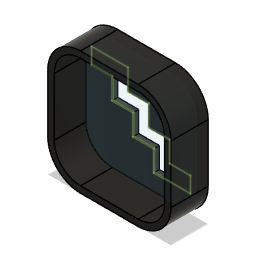
Trellis Keycap stairs (Autodesk Fusion 360 design; units mm, degrees)
Autodesk Fusion 360 part; units mm, degrees
sketch "Sketch1" plane through (0, 0, 0) normal (0, 0, 1) x (1, 0, 0)
  line L0 (2.72, 5) -> (-2.72, 5)
  line L1 (-5, 2.72) -> (-5, -2.72)
  line L2 (-2.72, -5) -> (2.72, -5)
  line L3 (5, -2.72) -> (5, 2.72)
  line L4 (5, 5) -> (-5, -5) construction
  line L5 (-5, 5) -> (5, -5) construction
  arc A0 (5, 2.72) -> (2.72, 5) centre (2.72, 2.72) ccw
  arc A1 (2.72, -5) -> (5, -2.72) centre (2.72, -2.72) ccw
  arc A2 (-5, -2.72) -> (-2.72, -5) centre (-2.72, -2.72) ccw
  arc A3 (-2.72, 5) -> (-5, 2.72) centre (-2.72, 2.72) ccw
  line L6 (-2.72, -5.2) -> (2.72, -5.2)
  arc A4 (2.72, -5.2) -> (5.2, -2.72) centre (2.72, -2.72) ccw
  line L7 (5.2, -2.72) -> (5.2, 2.72)
  arc A5 (5.2, 2.72) -> (2.72, 5.2) centre (2.72, 2.72) ccw
  line L8 (2.72, 5.2) -> (-2.72, 5.2)
  arc A6 (-2.72, 5.2) -> (-5.2, 2.72) centre (-2.72, 2.72) ccw
  line L9 (-5.2, 2.72) -> (-5.2, -2.72)
  arc A7 (-5.2, -2.72) -> (-2.72, -5.2) centre (-2.72, -2.72) ccw
  line L10 (-2.72, -5.8) -> (2.72, -5.8)
  arc A8 (2.72, -5.8) -> (5.8, -2.72) centre (2.72, -2.72) ccw
  line L11 (5.8, -2.72) -> (5.8, 2.72)
  arc A9 (5.8, 2.72) -> (2.72, 5.8) centre (2.72, 2.72) ccw
  line L12 (2.72, 5.8) -> (-2.72, 5.8)
  arc A10 (-2.72, 5.8) -> (-5.8, 2.72) centre (-2.72, 2.72) ccw
  line L13 (-5.8, 2.72) -> (-5.8, -2.72)
  arc A11 (-5.8, -2.72) -> (-2.72, -5.8) centre (-2.72, -2.72) ccw
  dimension "d1" = 10
  dimension "d2" = 10
  dimension "d3" = 2.28
  dimension "d4" = 0.2
  dimension "d5" = 0.8
  constraint horizontal L0
  constraint perpendicular L0 L1
  constraint parallel L0 L2
  constraint parallel L1 L3
  constraint coincident L4 origin
  constraint coincident L5 origin
  constraint coincident L4.start L0
  constraint coincident L4.start L3
  constraint tangent L0 A0
  constraint tangent L3 A0
  constraint coincident L5.end L3
  constraint coincident L5.end L2
  constraint tangent L3 A1
  constraint tangent L2 A1
  constraint equal A0 A1
  constraint coincident L4.end L2
  constraint coincident L4.end L1
  constraint tangent L2 A2
  constraint tangent L1 A2
  constraint equal A0 A2
  constraint coincident L5.start L1
  constraint coincident L5.start L0
  constraint tangent L1 A3
  constraint tangent L0 A3
  constraint equal A0 A3
  measures "d1" distance of L4.end L5.end
  measures "d2" distance of L5.start L4.end
  measures "d3" radius of A0
extrude "Extrude1" add sketch "Sketch1" along normal blind 3 contours L10 A8 L11 A9 L12 A10 L13 A11 makes body 1
extrude "Extrude2" add sketch "Sketch1" against normal blind 0.5 contours L0 L1 L2 L3 A0 A1 A2 A3 | L6 A4 L7 A5 L8 A6 L9 A7 | L10 A8 L11 A9 L12 A10 L13 A11 bodies 1
sketch "Sketch2" plane through (0, 0, 0) normal (0, 0, 1) x (1, 0, 0)
  line L0 (-2.72, -5.2) -> (2.72, -5.2)
  arc A0 (2.72, -5.2) -> (5.2, -2.72) centre (2.72, -2.72) ccw
  line L1 (5.2, -2.72) -> (5.2, 2.72)
  arc A1 (5.2, 2.72) -> (2.72, 5.2) centre (2.72, 2.72) ccw
  line L2 (2.72, 5.2) -> (-2.72, 5.2)
  arc A2 (-2.72, 5.2) -> (-5.2, 2.72) centre (-2.72, 2.72) ccw
  line L3 (-5.2, 2.72) -> (-5.2, -2.72)
  arc A3 (-5.2, -2.72) -> (-2.72, -5.2) centre (-2.72, -2.72) ccw
  line L4 (-1.246, 3.6964) -> (-1.246, 1.7361)
  line L5 (-1.246, 1.7361) -> (0.7143, 1.7361)
  line L6 (0.7143, 1.7361) -> (0.7143, -0.2242)
  line L7 (0.7143, -0.2242) -> (2.6746, -0.2242)
  line L8 (2.6746, -0.2242) -> (2.6746, -2.1845)
  line L9 (2.6746, -2.1845) -> (4.6349, -2.1845)
  line L10 (4.6349, -2.1845) -> (4.6349, -3.6547)
  line L11 (4.6349, -3.6547) -> (1.2043, -3.6547)
  line L12 (1.2043, -3.6547) -> (1.2043, -1.6944)
  line L13 (1.2043, -1.6944) -> (-0.756, -1.6944)
  line L14 (-0.756, -1.6944) -> (-0.756, 0.2659)
  line L15 (-0.756, 0.2659) -> (-2.7163, 0.2659)
  line L16 (-2.7163, 0.2659) -> (-2.7163, 2.2262)
  line L17 (-2.7163, 2.2262) -> (-4.6766, 2.2262)
  line L18 (-4.6766, 2.2262) -> (-4.6766, 3.6964)
  line L19 (-4.6766, 3.6964) -> (-1.246, 3.6964)
extrude "Extrude3" cut sketch "Sketch2" against normal blind 0.5 contours L4 L5 L6 L7 L8 L9 L10 L11 L12 L13 L14 L15 L16 L17 L18 L19 bodies 1
extrude "Extrude4" add sketch "Sketch2" against normal blind 0.5 separate body contours L4 L5 L6 L7 L8 L9 L10 L11 L12 L13 L14 L15 L16 L17 L18 L19 makes body 2
named bodies: "Keycap"
